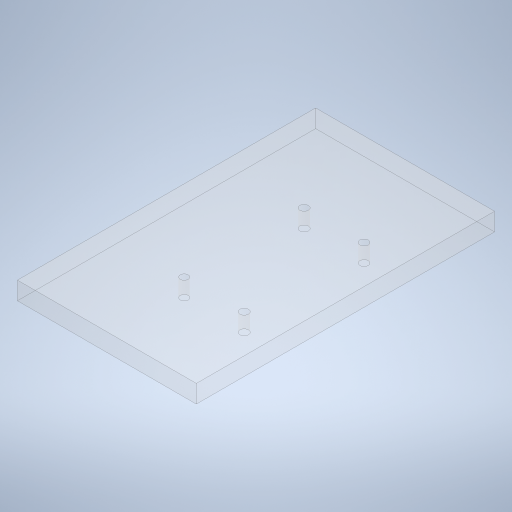
# Autodesk Inventor part: feet
Saved by Autodesk Inventor 2024 (Build 280153000, 153)
## iProperties
Created: 2024-09-08
Part Number: feet
Material: PMMA 플라스틱
Document SubType Name: Modeling
Designer: jmha0
Density: 1.188 g/cm^3
Appearance: 폴리카보네이트 - 선명
Author: jmha0
Autodesk Inventor part; units mm, degrees
ref_plane "YZ Plane" through (0, 0, 0) normal (1, 0, 0) x (0, 1, 0)
ref_plane "XZ Plane" through (0, 0, 0) normal (0, 1, 0) x (-1, 0, 0)
ref_plane "XY Plane" through (0, 0, 0) normal (0, 0, 1) x (1, 0, 0)
sketch "스케치1" plane through (0, 0, 0) normal (0, 1, 0) x (-1, 0, 0)
  line L0 (-5.3697, -35.4212) -> (-5.3697, -37.6212)
  line L1 (-5.3697, -37.6212) -> (-10.5697, -37.6212)
  line L2 (-10.5697, -37.6212) -> (-10.5697, -35.4212)
  line L3 (-10.5697, -35.4212) -> (-5.3697, -35.4212)
  line L4 (10.6803, 36.7788) -> (10.6803, 38.9788)
  line L5 (10.6803, 38.9788) -> (14.7303, 38.9788)
  line L6 (14.7303, 38.9788) -> (14.7303, 36.7788)
  line L7 (14.7303, 36.7788) -> (10.6803, 36.7788)
  line L8 (14.7303, -35.4212) -> (14.7303, -37.6212)
  line L9 (14.7303, -37.6212) -> (9.5303, -37.6212)
  line L10 (9.5303, -37.6212) -> (9.5303, -35.4212)
  line L11 (9.5303, -35.4212) -> (14.7303, -35.4212)
  line L12 (-5.3697, 36.7788) -> (-10.5697, 36.7788)
  line L13 (-10.5697, 36.7788) -> (-10.5697, 38.9788)
  line L14 (-10.5697, 38.9788) -> (-5.3697, 38.9788)
  line L15 (-5.3697, 38.9788) -> (-5.3697, 36.7788)
  circle A0 centre (12.1303, -19.4212) radius 1.45
  circle A1 centre (-7.9697, -19.4212) radius 1.45
  circle A2 centre (12.1303, 20.7788) radius 1.45
  circle A3 centre (-7.9697, 20.7788) radius 1.45
  line L16 (22.1803, -39.5212) -> (-18.0197, -39.5212)
  line L17 (22.1803, 40.8788) -> (22.1803, -39.5212)
  line L18 (-18.0197, 40.8788) -> (22.1803, 40.8788)
  line L19 (-18.0197, -39.5212) -> (-18.0197, 40.8788)
  line L20 (-27.9197, 50.6788) -> (32.0803, 50.6788)
  line L21 (32.0803, 50.6788) -> (32.0803, -49.3212)
  line L22 (32.0803, -49.3212) -> (-27.9197, -49.3212)
  line L23 (-27.9197, -49.3212) -> (-27.9197, 50.6788)
  line L24 (-27.9197, 50.6788) -> (32.0803, -49.3212) construction
  line L25 (32.0803, 50.6788) -> (-27.9197, -49.3212) construction
  circle A4 centre (12.1303, -19.4212) radius 1.35
  circle A5 centre (-7.9697, -19.4212) radius 1.35
  circle A6 centre (-7.9697, 20.7788) radius 1.35
  circle A7 centre (12.1303, 20.7788) radius 1.35
  circle A8 centre (2.0803, 0.6788) radius 4.7553
  point P0 (0, 0)
  dimension "d0" = 60
  dimension "d1" = 100
  dimension "d4" = 2.7
  dimension "d5" = 2.7
  dimension "d6" = 2.7
  dimension "d7" = 2.7
  constraints: 52 end point, 9 centre point, 5 coincident, 2 midpoint, 2 parallel, 1 horizontal, 1 perpendicular
  measures "d0" distance of L21.end L22.end
  measures "d1" distance of L20.end L21.end
  measures "d4" diameter of A4
  measures "d5" diameter of A5
  measures "d6" diameter of A6
  measures "d7" diameter of A7
extrude "돌출1" add sketch "스케치1" along normal blind 6 contours L0 L1 L2 L3 | L4 L5 L6 L7 | L8 L9 L10 L11 | L12 L13 L14 L15 | A0 | A1 | A2 | A3 | L16 L19 L18 L17 | L20 L21 L22 L23 | A4 | A5 | A6 | A7 | A8
sketch "스케치2" plane through (0, 6, 0) normal (0, 1, 0) x (1, 0, 0)
  line L0 (27.9197, 49.3212) -> (-32.0803, 49.3212) projected
  line L1 (-32.0803, 49.3212) -> (-32.0803, -50.6788) projected
  line L2 (-32.0803, -50.6788) -> (27.9197, -50.6788) projected
  line L3 (27.9197, -50.6788) -> (27.9197, 49.3212) projected
  line L4 (58.4667, -26.0223) -> (58.4667, -28.2223)
  line L5 (58.4667, -28.2223) -> (53.2667, -28.2223)
  line L6 (53.2667, -28.2223) -> (53.2667, -26.0223)
  line L7 (53.2667, -26.0223) -> (58.4667, -26.0223)
  circle A0 centre (15.0977, -21.818) radius 1.45
  circle A1 centre (-5.0023, -21.818) radius 1.45
  line L8 (73.3667, -26.0223) -> (78.5667, -26.0223)
  line L9 (78.5667, -26.0223) -> (78.5667, -28.2223)
  line L10 (73.3667, -28.2223) -> (73.3667, -26.0223)
  line L11 (78.5667, -28.2223) -> (73.3667, -28.2223)
  line L12 (86.0167, -30.1223) -> (45.8167, -30.1223)
  line L13 (74.5167, 46.1777) -> (74.5167, 48.3777)
  line L14 (74.5167, 48.3777) -> (78.5667, 48.3777)
  line L15 (78.5667, 48.3777) -> (78.5667, 46.1777)
  line L16 (45.8167, -30.1223) -> (45.8167, 50.2777)
  line L17 (86.0167, 50.2777) -> (86.0167, -30.1223)
  circle A2 centre (-5.0023, 18.382) radius 1.45
  circle A3 centre (15.0977, 18.382) radius 1.45
  line L18 (58.4667, 46.1777) -> (53.2667, 46.1777)
  line L19 (45.8167, 50.2777) -> (86.0167, 50.2777)
  line L20 (53.2667, 46.1777) -> (53.2667, 48.3777)
  line L21 (53.2667, 48.3777) -> (58.4667, 48.3777)
  line L22 (58.4667, 48.3777) -> (58.4667, 46.1777)
  line L23 (78.5667, 46.1777) -> (74.5167, 46.1777)
  line L24 (-26.6842, 49.3212) -> (33.3158, 49.3212)
  line L25 (33.3158, 49.3212) -> (33.3158, -50.6788)
  line L26 (33.3158, -50.6788) -> (-26.6842, -50.6788)
  line L27 (-26.6842, -50.6788) -> (-26.6842, 49.3212)
  line L28 (-26.6842, 49.3212) -> (33.3158, -50.6788) construction
  line L29 (33.3158, 49.3212) -> (-26.6842, -50.6788) construction
  circle A4 centre (15.0977, -21.818) radius 1.35
  circle A5 centre (-5.0023, -21.818) radius 1.35
  circle A6 centre (-5.0023, 18.382) radius 1.35
  circle A7 centre (15.0977, 18.382) radius 1.35
  circle A8 centre (3.3158, -0.6788) radius 4.7553
  circle A9 centre (-2.0803, -0.6788) radius 10.0549
  line L30 (-6.7392, -0.6788) -> (3.3158, -0.6788)
  point P0 (0, 0)
  point P1 (2.9674, -2.3969)
  dimension "d8" = 60
  dimension "d9" = 100
  dimension "d10" = 2.7
  dimension "d11" = 2.7
  dimension "d12" = 2.7
  dimension "d13" = 2.7
  constraints: 54 end point, 10 centre point, 5 coincident, 2 horizontal, 2 midpoint, 2 parallel, 1 perpendicular
  measures "d8" distance of L25.end L26.end
  measures "d9" distance of L24.end L25.end
  measures "d10" diameter of A4
  measures "d11" diameter of A5
  measures "d12" diameter of A6
  measures "d13" diameter of A7
extrude "돌출2" cut sketch "스케치2" against normal blind 6 contours A0 | A2 | A3 | A4 | A5 | A6 | A7
